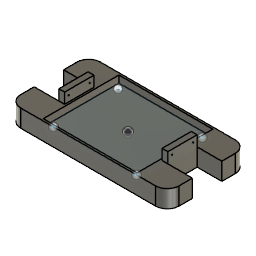
pendulo invertido (Autodesk Fusion 360 design; units mm, degrees)
Autodesk Fusion 360 part; units mm, degrees
sketch "Boceto1" plane through (0, 0, 0) normal (0, 0, 1) x (1, 0, 0)
  line L0 (57.5, 34) -> (-57.5, 34)
  line L1 (-67.5, 24) -> (-67.5, -24)
  line L2 (-57.5, -34) -> (57.5, -34)
  line L3 (67.5, -24) -> (67.5, 24)
  line L4 (67.5, 34) -> (-67.5, -34) construction
  line L5 (-67.5, 34) -> (67.5, -34) construction
  arc A0 (-57.5, 34) -> (-67.5, 24) centre (-57.5, 24) ccw
  arc A1 (-67.5, -24) -> (-57.5, -34) centre (-57.5, -24) ccw
  arc A2 (57.5, -34) -> (67.5, -24) centre (57.5, -24) ccw
  arc A3 (67.5, 24) -> (57.5, 34) centre (57.5, 24) ccw
  dimension "d1" = 135
  dimension "d2" = 68
  dimension "d3" = 10
  dimension "d4" = 10
  constraint horizontal L0
  constraint perpendicular L0 L1
  constraint parallel L0 L2
  constraint parallel L1 L3
  constraint coincident L4 origin
  constraint coincident L5 origin
  constraint coincident L5.start L0
  constraint coincident L5.start L1
  constraint tangent L0 A0
  constraint tangent L1 A0
  constraint coincident L4.end L1
  constraint coincident L4.end L2
  constraint tangent L1 A1
  constraint tangent L2 A1
  constraint equal A0 A1
  constraint coincident L5.end L2
  constraint coincident L5.end L3
  constraint tangent L2 A2
  constraint tangent L3 A2
  constraint equal A0 A2
  constraint coincident L4.start L3
  constraint coincident L4.start L0
  constraint tangent L3 A3
  constraint tangent L0 A3
  measures "d1" distance of L4.end L5.end
  measures "d2" distance of L5.start L4.end
  measures "d3" radius of A0
  measures "d4" radius of A3
extrude "Extruir1" add sketch "Boceto1" along normal blind 15
sketch "Boceto2" plane through (0, 0, 0) normal (0, 0, 1) x (1, 0, 0)
  line L0 (-46.5, 12.5) -> (-88.5, 12.5)
  line L1 (-88.5, 12.5) -> (-88.5, -12.5)
  line L2 (-88.5, -12.5) -> (-46.5, -12.5)
  line L3 (-46.5, -12.5) -> (-46.5, 12.5)
  line L4 (-46.5, 12.5) -> (-88.5, -12.5) construction
  line L5 (-88.5, 12.5) -> (-46.5, -12.5) construction
  point P0 (-67.5, 0)
  dimension "d7" = 42
  dimension "d8" = 25
  constraint horizontal L0
  constraint perpendicular L0 L1
  constraint parallel L0 L2
  constraint parallel L1 L3
  constraint coincident L4 P0
  constraint coincident L5 P0
  measures "d7" distance of L1.end L2.end
  measures "d8" distance of L0.end L1.end
extrude "Extruir2" cut sketch "Boceto2" along normal blind 20
sketch "Boceto3" plane through (0, 0, 0) normal (0, 0, 1) x (1, 0, 0)
  line L0 (46.5, 12.5) -> (88.5, 12.5)
  line L1 (88.5, 12.5) -> (88.5, -12.5)
  line L2 (88.5, -12.5) -> (46.5, -12.5)
  line L3 (46.5, -12.5) -> (46.5, 12.5)
  line L4 (46.5, 12.5) -> (88.5, -12.5) construction
  line L5 (88.5, 12.5) -> (46.5, -12.5) construction
  point P0 (67.5, 0)
  dimension "d11" = 42
  dimension "d12" = 25
  constraint horizontal L0
  constraint perpendicular L0 L1
  constraint parallel L0 L2
  constraint parallel L1 L3
  constraint coincident L4 P0
  constraint coincident L5 P0
  measures "d11" distance of L1.end L2.end
  measures "d12" distance of L0.end L1.end
extrude "Extruir3" cut sketch "Boceto3" along normal blind 20
sketch "Boceto4" plane through (0, 0, 15) normal (0, 0, 1) x (-1, 0, 0)
  line L0 (-46.5, -12.5) -> (-67.5, -12.5)
  line L1 (-67.5, -12.5) -> (-67.5, -24)
  arc A0 (-67.5, -24) -> (-57.5, -34) centre (-57.5, -24) ccw
  line L2 (-57.5, -34) -> (57.5, -34)
  arc A1 (57.5, -34) -> (67.5, -24) centre (57.5, -24) ccw
  line L3 (67.5, -24) -> (67.5, -12.5)
  line L4 (67.5, -12.5) -> (46.5, -12.5)
  line L5 (46.5, -12.5) -> (46.5, 12.5)
  line L6 (46.5, 12.5) -> (67.5, 12.5)
  line L7 (67.5, 12.5) -> (67.5, 24)
  arc A2 (67.5, 24) -> (57.5, 34) centre (57.5, 24) ccw
  line L8 (57.5, 34) -> (-57.5, 34)
  arc A3 (-57.5, 34) -> (-67.5, 24) centre (-57.5, 24) ccw
  line L9 (-67.5, 24) -> (-67.5, 12.5)
  line L10 (-67.5, 12.5) -> (-46.5, 12.5)
  line L11 (-46.5, 12.5) -> (-46.5, -12.5)
  line L12 (-40, -32.25) -> (40, -32.25)
  line L13 (40, -32.25) -> (40, 32.25)
  line L14 (40, 32.25) -> (-40, 32.25)
  line L15 (-40, 32.25) -> (-40, -32.25)
  line L16 (-40, -32.25) -> (40, 32.25) construction
  line L17 (40, -32.25) -> (-40, 32.25) construction
  dimension "d15" = 80
  dimension "d16" = 64.5
  constraint horizontal L12
  constraint perpendicular L12 L13
  constraint parallel L12 L14
  constraint parallel L13 L15
  constraint coincident L16 origin
  constraint coincident L17 origin
  measures "d15" distance of L13.end L14.end
  measures "d16" distance of L12.end L13.end
extrude "Extruir4" cut sketch "Boceto4" against normal blind 6 contours L12 L13 L14 L15
sketch "Boceto5" plane through (0, 0, 9) normal (0, 0, 1) x (-1, 0, 0)
  line L0 (-40, 32.25) -> (-40, -32.25)
  line L1 (-40, -32.25) -> (40, -32.25)
  line L2 (40, -32.25) -> (40, 32.25)
  line L3 (40, 32.25) -> (-40, 32.25)
  circle A0 centre (35.57, 28.05) radius 0.9
  circle A1 centre (-35.37, 28.05) radius 0.9
  circle A2 centre (36.07, -27.5291) radius 0.9
  circle A3 centre (-35.87, -27.5291) radius 0.9
  dimension "d23" = 1.8
  dimension "d25" = 1.8
  dimension "d29" = 1.8
  dimension "d30" = 1.8
  measures "d23" diameter of A0
  measures "d25" diameter of A1
  measures "d29" diameter of A2
  measures "d30" diameter of A3
extrude "Extruir5" cut sketch "Boceto5" against normal blind 10 contours A3
extrude "Extruir6" cut sketch "Boceto5" against normal blind 10 contours A2
extrude "Extruir7" cut sketch "Boceto5" against normal blind 10 contours A0
extrude "Extruir8" cut sketch "Boceto5" against normal blind 10 contours A1
sketch "Boceto6" plane through (0, 0, 15) normal (0, 0, 1) x (-1, 0, 0)
  line L0 (40, -32.25) -> (-40, -32.25)
  line L1 (-40, -32.25) -> (-40, 32.25)
  line L2 (-40, 32.25) -> (40, 32.25)
  line L3 (40, 32.25) -> (40, -32.25)
  line L4 (-46.5, -12.5) -> (-67.5, -12.5)
  line L5 (-67.5, -12.5) -> (-67.5, -24)
  arc A0 (-67.5, -24) -> (-57.5, -34) centre (-57.5, -24) ccw
  line L6 (-57.5, -34) -> (57.5, -34)
  arc A1 (57.5, -34) -> (67.5, -24) centre (57.5, -24) ccw
  line L7 (67.5, -24) -> (67.5, -12.5)
  line L8 (67.5, -12.5) -> (46.5, -12.5)
  line L9 (46.5, -12.5) -> (46.5, 12.5)
  line L10 (46.5, 12.5) -> (67.5, 12.5)
  line L11 (67.5, 12.5) -> (67.5, 24)
  arc A2 (67.5, 24) -> (57.5, 34) centre (57.5, 24) ccw
  line L12 (57.5, 34) -> (-57.5, 34)
  arc A3 (-57.5, 34) -> (-67.5, 24) centre (-57.5, 24) ccw
  line L13 (-67.5, 24) -> (-67.5, 12.5)
  line L14 (-67.5, 12.5) -> (-46.5, 12.5)
  line L15 (-46.5, 12.5) -> (-46.5, -12.5)
  line L16 (46.5, -12.5) -> (41.5383, -12.5)
  line L17 (41.5383, -12.5) -> (41.5383, 12.5165)
  line L18 (41.5383, 12.5165) -> (46.5, 12.5165)
  line L19 (46.5, 12.5165) -> (46.5, -12.5)
  constraint horizontal L16
  constraint vertical L17
  constraint horizontal L18
  constraint vertical L19
  constraint coincident L8.end L9.start
extrude "Extruir9" add sketch "Boceto6" along normal blind 22 contours L9 L16 L17 L18 L19
sketch "Boceto7" plane through (0, 0, 15) normal (0, 0, 1) x (-1, 0, 0)
  line L0 (46.5, -12.5) -> (41.5383, -12.5)
  line L1 (41.5383, -12.5) -> (41.5383, 12.5165)
  line L2 (41.5383, 12.5165) -> (46.5, 12.5165)
  line L3 (46.5, 12.5165) -> (46.5, 12.5)
  line L4 (46.5, 12.5) -> (67.5, 12.5)
  line L5 (67.5, 12.5) -> (67.5, 24)
  arc A0 (67.5, 24) -> (57.5, 34) centre (57.5, 24) ccw
  line L6 (57.5, 34) -> (-57.5, 34)
  arc A1 (-57.5, 34) -> (-67.5, 24) centre (-57.5, 24) ccw
  line L7 (-67.5, 24) -> (-67.5, 12.5)
  line L8 (-67.5, 12.5) -> (-46.5, 12.5)
  line L9 (-46.5, 12.5) -> (-46.5, -12.5)
  line L10 (-46.5, -12.5) -> (-67.5, -12.5)
  line L11 (-67.5, -12.5) -> (-67.5, -24)
  arc A2 (-67.5, -24) -> (-57.5, -34) centre (-57.5, -24) ccw
  line L12 (-57.5, -34) -> (57.5, -34)
  arc A3 (57.5, -34) -> (67.5, -24) centre (57.5, -24) ccw
  line L13 (67.5, -24) -> (67.5, -12.5)
  line L14 (67.5, -12.5) -> (46.5, -12.5)
  line L15 (40, -32.25) -> (-40, -32.25)
  line L16 (-40, -32.25) -> (-40, 32.25)
  line L17 (-40, 32.25) -> (40, 32.25)
  line L18 (40, 32.25) -> (40, -32.25)
  line L19 (-46.5, -12.5) -> (-41.538, -12.5)
  line L20 (-41.538, -12.5) -> (-41.538, 12.5)
  line L21 (-41.538, 12.5) -> (-46.5, 12.5)
  line L22 (-46.5, 12.5) -> (-46.5, -12.5)
  dimension "d41" = 4.962
  constraint horizontal L19
  constraint vertical L20
  constraint horizontal L21
  constraint vertical L22
  constraint coincident L9.end L10.start
  measures "d41" distance of L20 L22
extrude "Extruir10" add sketch "Boceto7" along normal blind 9 contours L9 L19 L20 L21 L22
sketch "Boceto8" plane through (0, 0, 37) normal (0, 0, 1) x (-1, 0, 0)
  line L0 (46.5, 12.5165) -> (41.5383, 12.5165)
  line L1 (41.5383, 12.5165) -> (41.5383, -12.5)
  line L2 (41.5383, -12.5) -> (46.5, -12.5)
  line L3 (46.5, -12.5) -> (46.5, 12.5165)
  line L4 (46.5, -12.5) -> (41.5383, -12.5)
  line L5 (41.5383, -12.5) -> (41.5383, 12.5165)
  line L6 (41.5383, 12.5165) -> (46.5, 12.5165)
  line L7 (46.5, 12.5165) -> (46.5, -12.5)
  constraint horizontal L4
  constraint vertical L5
  constraint horizontal L6
  constraint vertical L7
  constraint coincident L0.end L1.start
  constraint coincident L2.end L3.start
extrude "Extruir11" cut sketch "Boceto8" against normal blind 13
sketch "Boceto9" plane through (46.5, 0, 0) normal (1, 0, 0) x (0, 1, 0)
  line L0 (-12.5, 15) -> (-12.5, 0)
  line L1 (-12.5, 0) -> (12.5, 0)
  line L2 (12.5, 0) -> (12.5, 15)
  line L3 (12.5, 15) -> (12.5, 24)
  line L4 (12.5, 24) -> (-12.5, 24)
  line L5 (-12.5, 24) -> (-12.5, 15)
  circle A0 centre (-9, 18.5) radius 0.5
  circle A1 centre (9, 18.5) radius 0.5
  dimension "d51" = 1
  dimension "d52" = 1
  measures "d51" diameter of A0
  measures "d52" diameter of A1
extrude "Extruir12" cut sketch "Boceto9" against normal blind 10 contours A0
extrude "Extruir13" cut sketch "Boceto9" against normal blind 10 contours A1
sketch "Boceto10" plane through (-46.5, 0, 0) normal (-1, 0, 0) x (0, -1, 0)
  line L0 (12.5165, 24) -> (-12.5, 24)
  line L1 (-12.5, 24) -> (-12.5, 15)
  line L2 (-12.5, 15) -> (-12.5, 0)
  line L3 (-12.5, 0) -> (12.5, 0)
  line L4 (12.5, 0) -> (12.5, 15)
  line L5 (12.5, 15) -> (12.5165, 15)
  line L6 (12.5165, 15) -> (12.5165, 24)
  circle A0 centre (-9, 20) radius 0.5
  circle A1 centre (9, 20) radius 0.5
  dimension "d62" = 1
  dimension "d63" = 1
  measures "d62" diameter of A0
  measures "d63" diameter of A1
extrude "Extruir14" cut sketch "Boceto10" against normal blind 15 contours A0
extrude "Extruir15" cut sketch "Boceto10" against normal blind 15 contours A1
extrude "Extruir16" add sketch "Boceto9" against normal blind 6 contours A0
extrude "Extruir17" add sketch "Boceto9" against normal blind 5 contours A1
delete_face "SuprimirCaras1" 1 faces at (40.846, -9.4698, 18.329)
sketch "Boceto11" plane through (46.5, 0, 0) normal (1, 0, 0) x (0, 1, 0)
  line L0 (12.5, 24) -> (-12.5, 24)
  circle A0 centre (-9, 20) radius 0.5
  circle A1 centre (9, 20) radius 0.5
  dimension "d76" = 1
  dimension "d77" = 1
  measures "d76" diameter of A0
  measures "d77" diameter of A1
extrude "Extruir18" cut sketch "Boceto11" against normal blind 10 contours A0
extrude "Extruir19" cut sketch "Boceto11" against normal blind 13 contours A1
